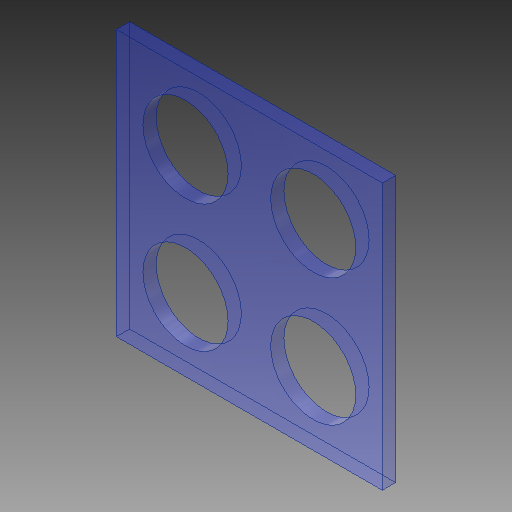
# Autodesk Inventor part: tank_front
Saved by Autodesk Inventor 2018.1 (Build 221171000, 171)
## iProperties
Created: 2017-07-30
Part Number: tank_front
Material: PVC-Piping
Document SubType Name: Modeling
Designer: Tom
Density: 1.4 g/cm^3
Appearance: Clear - Blue
Mass: 38.9613 g
Surface Area: 170.478 cm^2
Volume: 27.8295 cm^3
Author: Tom
Autodesk Inventor part; units mm, degrees
ref_plane "YZ Plane" through (0, 0, 0) normal (1, 0, 0) x (0, 1, 0)
ref_plane "XZ Plane" through (0, 0, 0) normal (0, 1, 0) x (-1, 0, 0)
ref_plane "XY Plane" through (0, 0, 0) normal (0, 0, 1) x (1, 0, 0)
sketch "Sketch1" plane through (0, 0, 0) normal (0, 0, 1) x (1, 0, 0)
  line L0 (0, 0) -> (100, 0)
  line L1 (100, 0) -> (100, 100)
  line L2 (100, 100) -> (0, 100)
  line L3 (0, 100) -> (0, 0)
  dimension "d0" = 100
  dimension "d1" = 100
  constraints: 8 end point, 2 parallel, 1 horizontal, 1 perpendicular
  measures "d0" distance of L2.end L1.end
  measures "d1" distance of L1.end L0.end
extrude "Extrusion1" add sketch "Sketch1" along normal blind 5
sketch "Sketch2" plane through (0, 0, 5) normal (0, 0, 1) x (1, 0, 0)
  line L0 (100, 100) -> (0, 100) construction
  line L1 (0, 0) -> (100, 0) construction
  line L2 (100, 0) -> (100, 100) construction
  line L3 (0, 100) -> (0, 0) construction
  circle A0 centre (26, 74) radius 16
  circle A1 centre (74, 26) radius 16
  circle A2 centre (74, 74) radius 16
  circle A3 centre (26, 26) radius 16
  dimension "d4" = 32
  dimension "d5" = 32
  dimension "d6" = 32
  dimension "d7" = 32
  dimension "d15" = 26
  dimension "d16" = 26
  dimension "d17" = 26
  dimension "d18" = 26
  dimension "d19" = 26
  dimension "d20" = 26
  dimension "d21" = 26
  dimension "d22" = 26
  dimension "d23" = 48
  dimension "d24" = 48
  dimension "d25" = 48
  dimension "d26" = 48
  constraints: 4 centre point
  measures "d4" diameter of A0
  measures "d5" diameter of A1
  measures "d6" diameter of A2
  measures "d7" diameter of A3
  measures "d15" distance from line of L3 A0.centre
  measures "d16" distance from line of L0 A0.centre
  measures "d17" distance from line of L0 A2.centre
  measures "d18" distance from line of L2 A2.centre
  measures "d19" distance from line of L2 A1.centre
  measures "d20" distance from line of L1 A1.centre
  measures "d21" distance from line of L1 A3.centre
  measures "d22" distance from line of L3 A3.centre
  measures "d23" distance of A2.centre A0.centre
  measures "d24" distance of A1.centre A2.centre
  measures "d25" distance of A3.centre A0.centre
  measures "d26" distance of A1.centre A3.centre
extrude "Extrusion3" cut sketch "Sketch2" against normal blind 5
equation "\"d0\" = tankw"
equation "\"d1\" = sensorsupportl"
equation "\"d2\" = pvct"
equation "\"d4\" = diahcl"
equation "\"d5\" = diaph"
equation "\"d6\" = diacucl"
equation "\"d7\" = diaetape"
equation "\"d15\" = 0.5 * diahcl + 2 * pvct"
equation "\"d16\" = 0.5 * diahcl + 2 * pvct"
equation "\"d17\" = 0.5 * diacucl + 2 * pvct"
equation "\"d18\" = 0.5 * diacucl + 2 * pvct"
equation "\"d19\" = 0.5 * diaph + 2 * pvct"
equation "\"d20\" = 0.5 * diaph + 2 * pvct"
equation "\"d21\" = 0.5 * diaetape + 2 * pvct"
equation "\"d22\" = 0.5 * diaetape + 2 * pvct"
equation "\"d29\" = pvct"
equation "\"lcsd\" = 19.05"
equation "\"lcwd1\" = 25"
equation "\"lcwd2\" = 34"
equation "\"lch1\" = 39"
equation "\"lcwd3\" = 43"
equation "\"dia1\" = 6"
equation "\"td\" = 18"
equation "\"bhh\" = 6"
equation "\"sw\" = 25"
equation "\"sh\" = 31"
equation "\"spacert\" = 2"
equation "\"pvct\" = 5"
equation "\"tankw\" = 100"
equation "\"tankl\" = 379"
equation "\"dia3\" = 8"
equation "\"dia4\" = 11"
equation "\"play\" = 9"
equation "\"holeh\" = 26"
equation "\"surroundt\" = 5"
equation "\"slack\" = 0.5"
equation "\"play2\" = 3"
equation "\"diaoverflow\" = 25"
equation "\"diacucl\" = 32"
equation "\"diawater\" = 25"
equation "\"diaph\" = 32"
equation "\"diaair\" = 32"
equation "\"diasurroundhole\" = 42"
equation "\"sensorsupportl\" = 100"
equation "\"diagrate\" = 12"
equation "\"gratespacing\" = 12.02082"
equation "\"sidedist\" = 13.9375"
equation "\"bottomdist\" = 9.6355"
equation "\"diahcl\" = 32"
equation "\"bracketwtop\" = 6"
equation "\"bracketwbottom\" = 6"
equation "\"nett\" = 1"
equation "\"nethole\" = 16"
equation "\"netside\" = 3.5"
equation "\"nettop\" = 7"
equation "\"netholespacing\" = 2"
equation "\"diaetape\" = 32"
body "Solid1"
